[a]_front_grill_logo_plates (Autodesk Fusion 360 design; units mm, degrees)
Autodesk Fusion 360 part; units mm, degrees
sketch "Sketch1" plane through (0, 0, 0) normal (0, 0, 1) x (1, 0, 0)
  line L0 (10, -25.5) -> (-10, -25.5)
  line L1 (-10, -25.5) -> (-10, 25.5)
  line L2 (-10, 25.5) -> (10, 25.5)
  line L3 (10, 25.5) -> (10, -25.5)
  line L4 (10, -25.5) -> (-10, 25.5) construction
  line L5 (-10, -25.5) -> (10, 25.5) construction
  spline S0 degree 3 poles (20.9021, -27.1092) (20.9021, -23.7596) (20.9021, -20.4205) (20.9021, -17.0656) knots 0 0 0 0 1 1 1 1
  spline S1 degree 3 poles (20.9021, -17.0656) (20.9815, -17.0656) (21.0502, -17.0656) (21.119, -17.0656) knots 0 0 0 0 1 1 1 1
  spline S2 degree 3 poles (21.119, -17.0656) (22.2144, -17.0656) (23.3151, -17.0603) (24.4105, -17.0656) knots 0 0 0 0 1 1 1 1
  spline S3 degree 3 poles (24.4105, -17.0656) (24.548, -17.0656) (24.6274, -17.0233) (24.6856, -16.9016) knots 0 0 0 0 1 1 1 1
  spline S4 degree 3 poles (24.6856, -16.9016) (24.765, -16.7375) (24.8655, -16.5841) (24.9449, -16.3989) knots 0 0 0 0 1 1 1 1
  spline S5 degree 3 poles (24.9449, -16.3989) (24.6962, -16.7217) (24.384, -16.8487) (24.0295, -16.7481) knots 0 0 0 0 1 1 1 1
  spline S6 degree 3 poles (24.0295, -16.7481) (24.6645, -16.1184) (25.3153, -15.4728) (25.945, -14.8484) knots 0 0 0 0 1 1 1 1
  spline S7 degree 3 poles (25.945, -14.8484) (26.5483, -15.4517) (27.1939, -16.0973) (27.8395, -16.7375) knots 0 0 0 0 1 1 1 1
  spline S8 degree 3 poles (27.8395, -16.7375) (27.4638, -16.8434) (27.1463, -16.727) (26.9187, -16.3671) knots 0 0 0 0 1 1 1 1
  spline S9 degree 3 poles (26.9187, -16.3671) (26.9081, -16.383) (26.8923, -16.3989) (26.8817, -16.4148) knots 0 0 0 0 1 1 1 1
  spline S10 degree 3 poles (26.8817, -16.4148) (26.9981, -16.6158) (27.1092, -16.8222) (27.2362, -17.0127) knots 0 0 0 0 1 1 1 1
  spline S11 degree 3 poles (27.2362, -17.0127) (27.2627, -17.055) (27.3632, -17.055) (27.432, -17.055) knots 0 0 0 0 1 1 1 1
  spline S12 degree 3 poles (27.432, -17.055) (28.5221, -17.055) (29.6122, -17.055) (30.7023, -17.055) knots 0 0 0 0 1 1 1 1
  spline S13 degree 3 poles (30.7023, -17.055) (30.771, -17.055) (30.8451, -17.055) (30.9298, -17.055) knots 0 0 0 0 1 1 1 1
  spline S14 degree 3 poles (30.9298, -17.055) (30.9298, -20.4047) (30.9298, -23.749) (30.9298, -27.0986) knots 0 0 0 0 1 1 1 1
  spline S15 degree 3 poles (30.9298, -27.0986) (27.596, -27.1092) (24.2623, -27.1092) (20.9021, -27.1092) knots 0 0 0 0 1 1 1 1
  spline S16 degree 3 poles (29.9508, -22.606) (29.9191, -22.5584) (29.8926, -22.5266) (29.8715, -22.4843) knots 0 0 0 0 1 1 1 1
  spline S17 degree 3 poles (29.8715, -22.4843) (28.9454, -20.8756) (28.0141, -19.267) (27.088, -17.6583) knots 0 0 0 0 1 1 1 1
  spline S18 degree 3 poles (27.088, -17.6583) (27.0245, -17.5472) (26.961, -17.4995) (26.8288, -17.4995) knots 0 0 0 0 1 1 1 1
  spline S19 degree 3 poles (26.8288, -17.4995) (26.2255, -17.5101) (25.6223, -17.5101) (25.0137, -17.4995) knots 0 0 0 0 1 1 1 1
  spline S20 degree 3 poles (25.0137, -17.4995) (24.8814, -17.4995) (24.8179, -17.5472) (24.7544, -17.653) knots 0 0 0 0 1 1 1 1
  spline S21 degree 3 poles (24.7544, -17.653) (24.0824, -18.8278) (23.4103, -19.9972) (22.733, -21.1667) knots 0 0 0 0 1 1 1 1
  spline S22 degree 3 poles (22.733, -21.1667) (22.4578, -21.6429) (22.1827, -22.1192) (21.8969, -22.606) knots 0 0 0 0 1 1 1 1
  spline S23 degree 3 poles (21.8969, -22.606) (21.7699, -22.5319) (21.6535, -22.4631) (21.5265, -22.389) knots 0 0 0 0 1 1 1 1
  spline S24 degree 3 poles (21.5265, -22.389) (22.4684, -20.7592) (23.3998, -19.14) (24.3364, -17.5154) knots 0 0 0 0 1 1 1 1
  spline S25 degree 3 poles (24.3364, -17.5154) (23.3151, -17.5154) (22.3308, -17.5154) (21.336, -17.5154) knots 0 0 0 0 1 1 1 1
  spline S26 degree 3 poles (21.336, -17.5154) (21.336, -20.574) (21.336, -23.622) (21.336, -26.6753) knots 0 0 0 0 1 1 1 1
  spline S27 degree 3 poles (21.336, -26.6753) (24.3946, -26.6753) (27.4426, -26.6753) (30.4959, -26.6753) knots 0 0 0 0 1 1 1 1
  spline S28 degree 3 poles (30.4959, -26.6753) (30.4959, -23.6114) (30.4959, -20.5634) (30.4959, -17.5154) knots 0 0 0 0 1 1 1 1
  spline S29 degree 3 poles (30.4959, -17.5154) (29.4958, -17.5154) (28.5115, -17.5154) (27.5061, -17.5154) knots 0 0 0 0 1 1 1 1
  spline S30 degree 3 poles (27.5061, -17.5154) (28.448, -19.1505) (29.3846, -20.7698) (30.3213, -22.389) knots 0 0 0 0 1 1 1 1
  spline S31 degree 3 poles (30.3213, -22.389) (30.1837, -22.4737) (30.0725, -22.5372) (29.9508, -22.606) knots 0 0 0 0 1 1 1 1
  spline S32 degree 3 poles (26.7494, -17.0709) (26.4636, -16.5788) (26.199, -16.1184) (25.9239, -15.6422) knots 0 0 0 0 1 1 1 1
  spline S33 degree 3 poles (25.9239, -15.6422) (25.6434, -16.129) (25.3788, -16.5894) (25.1037, -17.0709) knots 0 0 0 0 1 1 1 1
  spline S34 degree 3 poles (25.1037, -17.0709) (25.6646, -17.0709) (26.1885, -17.0709) (26.7494, -17.0709) knots 0 0 0 0 1 1 1 1
  spline S35 degree 3 poles (28.9401, -27.4373) (27.9241, -28.4533) (26.924, -29.4534) (25.9345, -30.443) knots 0 0 0 0 1 1 1 1
  spline S36 degree 3 poles (25.9345, -30.443) (24.9396, -29.4481) (23.9395, -28.4427) (22.9341, -27.4373) knots 0 0 0 0 1 1 1 1
  spline S37 degree 3 poles (22.9341, -27.4373) (24.9185, -27.4373) (26.924, -27.4373) (28.9401, -27.4373) knots 0 0 0 0 1 1 1 1
  spline S38 degree 3 poles (18.1345, -22.643) (18.9548, -21.8228) (19.775, -20.9973) (20.5899, -20.1771) knots 0 0 0 0 1 1 1 1
  spline S39 degree 3 poles (20.5899, -20.1771) (20.5899, -21.8122) (20.5899, -23.458) (20.5899, -25.1037) knots 0 0 0 0 1 1 1 1
  spline S40 degree 3 poles (20.5899, -25.1037) (19.7591, -24.2729) (18.9389, -23.4474) (18.1345, -22.643) knots 0 0 0 0 1 1 1 1
  spline S41 degree 3 poles (31.2526, -25.0825) (31.2526, -23.4474) (31.2526, -21.8017) (31.2526, -20.1824) knots 0 0 0 0 1 1 1 1
  spline S42 degree 3 poles (31.2526, -20.1824) (32.0622, -21.0026) (32.8877, -21.8281) (33.6973, -22.643) knots 0 0 0 0 1 1 1 1
  spline S43 degree 3 poles (33.6973, -22.643) (32.9142, -23.4315) (32.0834, -24.257) (31.2526, -25.0825) knots 0 0 0 0 1 1 1 1
  line L6 (20.9021, -17.0656) -> (21.3413, -17.5207)
  line L7 (21.3413, -17.5207) -> (21.7752, -17.9546)
  line L8 (30.9351, -17.0656) -> (30.5012, -17.5207)
  line L9 (30.5012, -17.5207) -> (30.0831, -17.9388)
  line L10 (30.9351, -27.1145) -> (30.5012, -26.6806)
  line L11 (30.5012, -26.6806) -> (30.0673, -26.2467)
  line L12 (20.9021, -27.1092) -> (21.3413, -26.6806)
  line L13 (21.3413, -26.6806) -> (22.0451, -25.9768)
  line L14 (25.9239, -16.9757) -> (25.9239, -17.7959)
  line L15 (37.9475, 0.7379) -> (27.9475, 0.7379)
  line L16 (27.9475, 0.7379) -> (27.9475, 10.7379)
  line L17 (27.9475, 10.7379) -> (37.9475, 10.7379)
  line L18 (37.9475, 10.7379) -> (37.9475, 0.7379)
  line L19 (37.9475, 0.7379) -> (27.9475, 10.7379) construction
  line L20 (27.9475, 0.7379) -> (37.9475, 10.7379) construction
  line L21 (28.9475, 9.7379) -> (36.9475, 9.7379)
  line L22 (36.9475, 9.7379) -> (36.9475, 1.7379)
  line L23 (36.9475, 1.7379) -> (28.9475, 1.7379)
  line L24 (28.9475, 1.7379) -> (28.9475, 9.7379)
  line L25 (32.9475, 5.7379) -> (24.3475, 5.7379) construction
  line L26 (24.3475, 5.7379) -> (27.1475, 8.5379)
  line L27 (27.1475, 8.5379) -> (27.1475, 2.9379)
  line L28 (27.1475, 2.9379) -> (24.3475, 5.7379)
  line L29 (32.9475, 5.7379) -> (32.9475, 10.7379) construction
  line L30 (41.5475, 5.7379) -> (38.7475, 8.5379)
  line L31 (38.7475, 8.5379) -> (38.7475, 2.9379)
  line L32 (38.7475, 2.9379) -> (41.5475, 5.7379)
  line L33 (32.9475, 5.7379) -> (32.9475, -2.8621) construction
  line L34 (32.9475, -2.8621) -> (30.1475, -0.0621)
  line L35 (30.1475, -0.0621) -> (35.7475, -0.0621)
  line L36 (35.7475, -0.0621) -> (32.9475, -2.8621)
  line L37 (32.9475, 14.3379) -> (30.1475, 11.5379)
  line L38 (30.1475, 11.5379) -> (35.7475, 11.5379) construction
  line L39 (35.7475, 11.5379) -> (32.9475, 14.3379)
  line L40 (32.9475, 14.3379) -> (32.9475, 11.5379) construction
  line L41 (32.9475, 13.5379) -> (29.5411, 7.6379)
  line L42 (29.5411, 7.6379) -> (30.2339, 7.2379)
  line L43 (30.2339, 7.2379) -> (32.9475, 11.9379)
  line L44 (21.5265, -22.389) -> (24.9449, -16.3989)
  line L45 (25.945, -14.8484) -> (24.0295, -16.7481)
  line L46 (32.9475, 13.5379) -> (36.3539, 7.6379)
  line L47 (36.3539, 7.6379) -> (35.661, 7.2379)
  line L48 (35.661, 7.2379) -> (32.9475, 11.9379)
  arc A0 (30.1475, 11.5379) -> (32.2547, 12.3379) centre (30.1475, 14.713) ccw
  arc A1 (33.6403, 12.3379) -> (35.7475, 11.5379) centre (35.7475, 14.713) ccw
  arc A2 (-2.5, 5.2) -> (-0.5196, 6) centre (-2.5, 8.0512) ccw
  line L49 (-4, -4) -> (4, 4) construction
  line L50 (0, 6.9) -> (2.8868, 1.9)
  line L51 (0, 0) -> (0, -7.7) construction
  line L52 (7.7, 0) -> (5.2, 2.5)
  line L53 (-5.2, -2.5) -> (-7.7, 0)
  line L54 (-2.5, 5.2) -> (2.5, 5.2) construction
  line L55 (2.8868, 1.9) -> (2.3671, 1.6)
  arc A3 (0.5196, 6) -> (2.5, 5.2) centre (2.5, 8.0512) ccw
  line L56 (-4, -4) -> (-4, 4)
  line L57 (3.4, -3.4) -> (-3.4, -3.4)
  line L58 (-7.7, 0) -> (-5.2, 2.5)
  line L59 (3.4, 3.4) -> (3.4, -3.4)
  line L60 (0, -7.7) -> (-2.5, -5.2)
  line L61 (4, -4) -> (-4, -4)
  line L62 (0, 0) -> (0, 4) construction
  line L63 (4, -4) -> (-4, 4) construction
  line L64 (5.2, 2.5) -> (5.2, -2.5)
  line L65 (0, 6.9) -> (-2.8868, 1.9)
  line L66 (2.5, 5.2) -> (0, 7.7)
  line L67 (-3.4, 3.4) -> (3.4, 3.4)
  line L68 (4, 4) -> (4, -4)
  line L69 (-4, 4) -> (4, 4)
  line L70 (2.5, -5.2) -> (0, -7.7)
  line L71 (-2.3671, 1.6) -> (0, 5.7)
  line L72 (2.3671, 1.6) -> (0, 5.7)
  line L73 (0, 7.7) -> (0, 5.2) construction
  line L74 (-2.5, -5.2) -> (2.5, -5.2)
  line L75 (0, 7.7) -> (-2.5, 5.2)
  line L76 (-5.2, 2.5) -> (-5.2, -2.5)
  line L77 (-3.4, -3.4) -> (-3.4, 3.4)
  line L78 (-2.8868, 1.9) -> (-2.3671, 1.6)
  line L79 (0, 0) -> (-7.7, 0) construction
  line L80 (5.2, -2.5) -> (7.7, 0)
  line L81 (-5, 9) -> (-5, -9) construction
  circle A4 centre (-5, -9) radius 5 construction
  circle A5 centre (-5, 9) radius 3
  circle A6 centre (-5, 9) radius 1.7
  circle A7 centre (-5, -9) radius 3
  circle A8 centre (-5, -9) radius 1.7
  point P0 (32.9475, 5.7379)
  point P1 (-5, 0)
  dimension "d1" = 20
  dimension "d2" = 51
  dimension "d3" = 10
  dimension "d4" = 1
  dimension "d5" = 2.8
  dimension "d6" = 0.8
  dimension "d7" = 15
  dimension "d8" = 0.8
  dimension "d9" = 0.8
  dimension "d10" = 2.5
  dimension "d11" = 0.8
  dimension "d12" = 0.6
  dimension "d13" = 8
  dimension "d14" = 2.5
  dimension "d15" = 1.2
  dimension "d16" = 15
  dimension "d17" = 0.6
  dimension "d18" = 0.8
  dimension "d19" = 1.8
  dimension "d20" = 0.8
  dimension "d36" = 18
  dimension "d37" = 10
  dimension "d39" = 6
  dimension "d40" = 3.4
  constraint horizontal L0
  constraint perpendicular L0 L1
  constraint parallel L0 L2
  constraint parallel L1 L3
  constraint coincident L4 L51.start
  constraint coincident L5 L51.start
  constraint coincident L51.start L62.start
  constraint horizontal L15
  constraint perpendicular L15 L16
  constraint parallel L15 L17
  constraint parallel L16 L18
  constraint coincident L19 P0
  constraint coincident L20 P0
  constraint equal L15 L16
  constraint coincident P0 L25.start
  constraint perpendicular L16 L25
  constraint perpendicular L26 L28
  constraint vertical L27
  constraint midpoint L17 L29.end
  constraint symmetric L25.end L29 L30.start
  constraint symmetric L26.end L29 L30.end
  constraint symmetric L27.end L29 L31.end
  constraint vertical L33
  constraint equal L25 L33
  constraint parallel L20 L26
  constraint parallel L19 L34
  constraint perpendicular L34 L36
  constraint horizontal L35
  constraint equal L27 L35
  constraint symmetric L25 L33.end L37.start
  constraint symmetric L25 L34.end L37.end
  constraint symmetric L25 L35.end L38.end
  constraint midpoint L38 L40.end
  constraint coincident L40 L41.start
  constraint coincident L40 L43.end
  constraint parallel L41 L43
  constraint perpendicular L41 L42
  constraint coincident S23.end S24.start
  constraint coincident S4.end S5.start
  constraint coincident S6.end S7.start
  constraint coincident S5.end S6.start
  constraint symmetric L40 L41.start L46.start
  constraint symmetric L40 L41.end L46.end
  constraint symmetric L40 L42.end L47.end
  constraint symmetric L40 L43.end L48.end
  constraint tangent L38 A0
  constraint coincident L37.end L38.start
  constraint coincident L41 A0.end
  constraint symmetric L29 A0.end A1.start
  constraint symmetric L29 L37.end L38.end
  constraint symmetric L29 A0 A1
  constraint horizontal L61
  constraint perpendicular L56 L61
  constraint parallel L61 L69
  constraint parallel L56 L68
  constraint coincident L51.start L63
  constraint coincident L51.start L49
  constraint equal L56 L61
  constraint perpendicular L56 L79
  constraint perpendicular L53 L58
  constraint vertical L76
  constraint midpoint L62.end L69
  constraint symmetric L52.start L53.end L62
  constraint symmetric L58.end L52.end L62
  constraint symmetric L64.end L53.start L62
  constraint vertical L51
  constraint equal L51 L79
  constraint parallel L49 L58
  constraint parallel L60 L63
  constraint perpendicular L60 L70
  constraint horizontal L74
  constraint equal L74 L76
  constraint symmetric L66.end L51.end L79
  constraint symmetric L60.end A2.start L79
  constraint symmetric L70.start L54.end L79
  constraint midpoint L73.end L54
  constraint coincident L50.start L73
  constraint coincident L71.end L73
  constraint parallel L65 L71
  constraint perpendicular L65 L78
  constraint symmetric L50.start L65.start L73
  constraint symmetric L50.end L65.end L73
  constraint symmetric L71.start L55.end L73
  constraint symmetric L71.end L72.end L73
  constraint tangent A2 L54
  constraint coincident A2.start L54.start
  constraint coincident A2.end L65
  constraint symmetric A2.end A3.start L62
  constraint symmetric A2.start L54.end L62
  constraint symmetric A2 A3 L62
  constraint vertical L81
  constraint coincident L81.end A4.centre
  constraint midpoint L81 P1
  constraint coincident L79 P1
  constraint tangent L1 A4
  constraint coincident L81.start A5.centre
  constraint concentric A5 A6
  constraint concentric A4 A7
  constraint concentric A7 A8
  constraint equal A6 A8
  constraint equal A5 A7
  measures "d1" distance of L1.end L2.end
  measures "d2" distance of L0.end L1.end
  measures "d3" distance of L15.start L15.end
  measures "d5" distance of L25.end L27
  measures "d6" distance of L16 L27
  measures "d7" angle of L37 L41
  measures "d8" distance of L41 L43
  measures "d9" distance of L37.start L41.start
  measures "d10" distance of L21 L42.end
  measures "d11" distance of L38 A0.end
  measures "d13" distance of L49.start L61.start
  measures "d14" distance of L53.end L76
  measures "d15" distance of L56 L76
  measures "d16" angle of L65 L75
  measures "d17" distance of L65 L71
  measures "d18" distance of L66.end L50.start
  measures "d19" distance of L71.start L67
  measures "d20" distance of A2.end L54
  measures "d36" distance of L81.start L81.end
  measures "d37" diameter of A4 S42.end
  measures "d39" diameter of A7 S42.end
  measures "d40" diameter of A8 S42.end
extrude "Extrude1" add sketch "Sketch1" against normal blind 5 contours L0 L1 L2 L3 | A2 L50 A3 L65 L66 L75 | L50 L65 L69 L71 L72 | L65 L67 L69 L71 | L50 L56 L57 L59 L61 L65 L67 L68 L69 L77 | L65 L67 L71 L78 | L50 L55 L57 L59 L65 L67 L71 L72 L77 L78 | L69 L71 L72 | L67 L69 L71 L72 | L50 L67 L69 L72 | L50 L55 L67 L72 | L52 L64 L80 | L53 L58 L76 | L60 L70 L74 | A5 | A6 | A7 | A8 makes body 1
fillet "Fillet1" radius 2 4 edges at (-10, -25.5, -2.5) (-10, 25.5, -2.5) (10, -25.5, -2.5) (10, 25.5, -2.5) on bodies 1
sketch "Sketch2" plane through (0, 0, 0) normal (0, 0, 1) x (-1, 0, 0)
  arc A0 (-10, -23.5) -> (-8, -25.5) centre (-8, -23.5) ccw
  line L0 (-8, -25.5) -> (8, -25.5)
  arc A1 (8, -25.5) -> (10, -23.5) centre (8, -23.5) ccw
  line L1 (10, -23.5) -> (10, 23.5)
  arc A2 (10, 23.5) -> (8, 25.5) centre (8, 23.5) ccw
  line L2 (8, 25.5) -> (-8, 25.5)
  arc A3 (-8, 25.5) -> (-10, 23.5) centre (-8, 23.5) ccw
  line L3 (-10, 23.5) -> (-10, -23.5)
  line L4 (8, 24.7) -> (-8, 24.7)
  arc A4 (-8, 24.7) -> (-9.2, 23.5) centre (-8, 23.5) ccw
  line L5 (-9.2, 23.5) -> (-9.2, -23.5)
  arc A5 (-9.2, -23.5) -> (-8, -24.7) centre (-8, -23.5) ccw
  line L6 (-8, -24.7) -> (8, -24.7)
  arc A6 (8, -24.7) -> (9.2, -23.5) centre (8, -23.5) ccw
  line L7 (9.2, -23.5) -> (9.2, 23.5)
  arc A7 (9.2, 23.5) -> (8, 24.7) centre (8, 23.5) ccw
  line L8 (8.6, -23.5) -> (8.6, 23.5)
  arc A8 (8.6, 23.5) -> (8, 24.1) centre (8, 23.5) ccw
  line L9 (8, 24.1) -> (-8, 24.1)
  arc A9 (-8, 24.1) -> (-8.6, 23.5) centre (-8, 23.5) ccw
  line L10 (-8.6, 23.5) -> (-8.6, -23.5)
  arc A10 (-8.6, -23.5) -> (-8, -24.1) centre (-8, -23.5) ccw
  line L11 (-8, -24.1) -> (8, -24.1)
  arc A11 (8, -24.1) -> (8.6, -23.5) centre (8, -23.5) ccw
  dimension "d27" = -0.8
  dimension "d29" = -0.6
extrude "Extrude3" cut sketch "Sketch2" against normal blind 1 contours A0 L0 A1 L1 A2 L2 A3 L3 bodies 1
extrude "Extrude2" cut sketch "Sketch1" against normal blind 0.8 contours A2 L50 A3 L65 L66 L75 | L50 L65 L69 L71 L72 | L65 L67 L69 L71 | L50 L56 L57 L59 L61 L65 L67 L68 L69 L77 | L65 L67 L71 L78 | L67 L69 L71 L72 | L50 L67 L69 L72 | L50 L55 L67 L72 | L52 L64 L80 | L53 L58 L76 | L60 L70 L74 bodies 1
fillet "Fillet2" radius 0.6 8 edges at (-10, 0, -1) (-9.4142, 24.9142, -1) (0, 25.5, -1) (9.4142, 24.9142, -1) (10, 0, -1) (9.4142, -24.9142, -1) (0, -25.5, -1) (-9.4142, -24.9142, -1) on bodies 1
fillet "Fillet3" radius 0.4 8 edges at (0, -24.7, 0) (8.8485, -24.3485, 0) (9.2, 0, 0) (8.8485, 24.3485, 0) (0, 24.7, 0) (-8.8485, 24.3485, 0) (-9.2, 0, 0) (-8.8485, -24.3485, 0) on bodies 1
extrude "Extrude4" cut sketch "Sketch1" against normal blind 5 contours A6 | A8 bodies 1
extrude "Extrude5" cut sketch "Sketch1" against normal blind 3 contours A5 | A7 bodies 1
chamfer "Chamfer1" distance 0.2 angle 45 4 edges at (-7.797, -7.9152, 0) (-7.797, 10.0848, 0) (-6.585, 8.3853, -3) (-6.585, -9.6147, -3) measured on face at (-1.3013, -20.1309, 0) measured on face at (-1.3013, -20.1309, 0) measured on face at (-3.3084, 8.8307, -3.6667) measured on face at (-3.3084, -9.1693, -3.6667) on bodies 1
chamfer "Chamfer2" distance 0.4 angle 45 1 faces at (5.5415, -2.833, -5) on bodies 1
mirror "Mirror1" about plane through (0, 0, 0) normal (1, 0, 0) of bodies 1 makes body 2
move_body "Move1" bodies 1 to x (1, 0, 0) y (0, 1, 0) z (0, 0, 1) at (-11, 0, 5)
move_body "Move2" bodies 2 to x (1, 0, 0) y (0, 1, 0) z (0, 0, 1) at (11, 0, 5)
equation "d4 = d3 * 0.1"
equation "d5 = d3 * 0.28"
equation "d6 = d3 * 0.08"
equation "d8 = d3 * 0.08"
equation "d9 = d8"
equation "d10 = d3 * 0.25"
equation "d11 = d9"
equation "d12 = d3 * 0.06"
equation "d14 = d3 * 0.25"
equation "d15 = d3 * 0.12"
equation "d17 = d3 * 0.06"
equation "d18 = d8"
equation "d19 = d3 * 0.18"
equation "d20 = d9"
